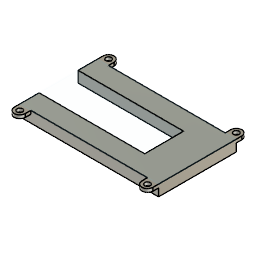
SMPS Stand (Autodesk Fusion 360 design; units mm, degrees)
part number: 2025-10-24-15-01-54-718
Autodesk Fusion 360 part; units mm, degrees
sketch "Sketch1" plane through (0, 0, 0) normal (0, 0, 1) x (1, 0, 0)
  line L0 (62.5, -35) -> (-62.5, -35)
  line L1 (-62.5, -35) -> (-62.5, 35)
  line L2 (-62.5, 35) -> (62.5, 35)
  line L3 (62.5, 35) -> (62.5, -35)
  line L4 (62.5, -35) -> (-62.5, 35) construction
  line L5 (-62.5, -35) -> (62.5, 35) construction
  dimension "d1" = 125
  dimension "d2" = 70
  constraint horizontal L0
  constraint perpendicular L0 L1
  constraint parallel L0 L2
  constraint parallel L1 L3
  constraint coincident L4 origin
  constraint coincident L5 origin
  measures "d1" distance of L1.end L2.end
  measures "d2" distance of L0.end L1.end
extrude "Extrude1" add sketch "Sketch1" along normal blind 10
sketch "Sketch2" plane through (0, 0, 10) normal (0, 0, 1) x (-1, 0, 0)
  line L0 (-62.5, -35) -> (62.5, -35)
  line L1 (62.5, -35) -> (62.5, 35)
  line L2 (62.5, 35) -> (-62.5, 35)
  line L3 (-62.5, 35) -> (-62.5, -35)
sketch "Sketch3" plane through (0, 0, 0) normal (0, 0, -1) x (1, 0, 0)
  line L0 (-62.5, -35) -> (62.5, -35)
  line L1 (62.5, -35) -> (62.5, 35)
  line L2 (62.5, 35) -> (-62.5, 35)
  line L3 (-62.5, 35) -> (-62.5, -35)
  line L4 (-62.5, 0) -> (-62.5, 17.5)
  line L5 (-62.5, 0) -> (-62.5, -17.5)
  line L6 (-62.5, 17.5) -> (32.5, 17.5)
  line L7 (32.5, 17.5) -> (32.5, -17.5)
  line L8 (-62.5, -17.5) -> (32.5, -17.5)
  dimension "d5" = 17.5
  dimension "d6" = 17.5
  dimension "d7" = 95
  dimension "d8" = 35
  constraint midpoint L3 L4.start
  constraint parallel L3 L4
  constraint parallel L3 L5
  constraint perpendicular L3 L6
  constraint perpendicular L6 L7
  measures "d5" distance of L4.start L4.end
  measures "d6" distance of L4.start L5.end
  measures "d7" distance of L4.end L6.end
  measures "d8" distance of L6.end L7.end
extrude "Extrude2" cut sketch "Sketch3" against normal blind 8 contours L3 L4 L5 L6 L7 L8
extrude "Extrude3" cut 1 faces at (-30.8333, -5.8333, 8) along direction (0, 0, 1) blind 30
sketch "Sketch4" plane through (0, 0, 10) normal (0, 0, 1) x (-1, 0, 0)
  line L0 (62.5, -35) -> (52.5, -35)
  line L1 (52.5, -35) -> (52.5, -40)
  line L2 (62.5, -40) -> (62.5, -35)
  arc A0 (57.5, -45) -> (62.5, -40) centre (57.5, -40) ccw
  arc A1 (52.5, -40) -> (57.5, -45) centre (57.5, -40) ccw
  circle A2 centre (57.5, -40) radius 2.5
  point P0 (62.5, -45)
  dimension "d13" = 10
  dimension "d14" = 10
  dimension "d15" = 5
  dimension "d16" = 5
  dimension "d17" = 5
  constraint horizontal L0
  constraint vertical L1
  constraint vertical L2
  constraint coincident P0 L2
  constraint tangent L2 A0
  constraint tangent L1 A1
  constraint coincident A0.start A1.end
  constraint concentric A0 A2
  measures "d13" distance of L0.start L0.end
  measures "d14" distance of L0.start P0
  measures "d15" radius of A0
  measures "d16" radius of A1
  measures "d17" diameter of A2
extrude "Extrude4" add sketch "Sketch4" against normal blind 3
mirror "Mirror1" about plane through (0, 0, 0) normal (1, 0, 0) of "Extrude4"
mirror "Mirror2" about plane through (0, 0, 0) normal (0, 1, 0) of "Extrude4", "Mirror1"
equation "d5 = ( 35 / 2 ) * 1 mm"
